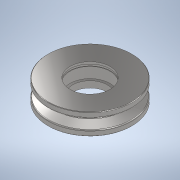
# Autodesk Inventor part: Pully
Saved by Autodesk Inventor 2021.1 (Build 251245010, 245A)
## iProperties
Created: 2025-09-16
Part Number: Pully
Material: Steel, Cast
Document SubType Name: Modeling
Designer: SD
Density: 7.85 g/cm^3
Appearance: Semi-Polished
Mass: 64.3377 g
Surface Area: 45.0663 cm^2
Volume: 8.19588 cm^3
Project: Automatic Tea Steeping mechanism
Length: 10.000 mm
BOM-Mass: 0.06434
BOM-Area: 0.005
Diameter: 40.000 mm
Author: SD
Title: Pully
Autodesk Inventor part; units mm, degrees
ref_plane "YZ Plane" through (0, 0, 0) normal (1, 0, 0) x (0, 1, 0)
ref_plane "XZ Plane" through (0, 0, 0) normal (0, 1, 0) x (-1, 0, 0)
ref_plane "XY Plane" through (0, 0, 0) normal (0, 0, 1) x (1, 0, 0)
sketch "Sketch1" plane through (0, 0, 0) normal (0, 0, 1) x (1, 0, 0)
  line L0 (0, 0) -> (0, -10) construction
  line L1 (8.25, -10) -> (20, -10)
  line L2 (20, -10) -> (20, -7.5)
  line L3 (20, -7.5) -> (15.3441, -5.75)
  line L4 (15.3441, -5.75) -> (15.3441, -4.25)
  line L5 (15.3441, -4.25) -> (20, -2.5)
  line L6 (20, -2.5) -> (20, 0)
  line L7 (20, 0) -> (9.5, 0)
  line L8 (9.5, 0) -> (9.5, -0.99)
  line L9 (9.5, -0.99) -> (9.8, -0.99)
  line L10 (9.8, -0.99) -> (9.8, -1.99)
  line L11 (9.8, -1.99) -> (9.5, -1.99)
  line L12 (9.5, -1.99) -> (9.5, -7)
  line L13 (9.5, -7) -> (8.25, -7)
  line L14 (8.25, -7) -> (8.25, -10)
  line L15 (15.3441, -5) -> (20.953, -5) construction
  dimension "d0" = 11.75
  dimension "d1" = 3
  dimension "Length" = 10
  dimension "d3" = 0.99
  dimension "d4" = 1
  dimension "d5" = 0.3
  dimension "d6" = 1.25
  dimension "d7" = 8.25
  dimension "d8" = 1.5
  dimension "d9" = 2.5
  dimension "d10" = 4.6559
  constraints: 32 end point, 8 perpendicular, 4 point on line, 2 equal length, 2 horizontal, 2 horizontal alignment, 1 midpoint, 1 parallel, 1 vertical
  measures "d0" distance of L1.start L1.end
  measures "d1" distance of L13.end L1.start
  measures "Length" distance between parallel lines of L7 L1
  measures "d3" distance of L7.end L8.end
  measures "d4" distance of L9.end L10.end
  measures "d5" distance of L8.end L9.end
  measures "d6" distance of L12.end L13.end
  measures "d7" distance between parallel lines of L14 L0
  measures "d8" distance of L3.end L4.end
  measures "d9" distance from line of L5.end L15
  measures "d10" distance between parallel lines of L6 L4
revolve "Revolution1" add sketch "Sketch1" angle 360 about axis through (0, 0, 0) along (0, -1, 0)
fillet "Fillet1" radius 0.5 4 edges at (-15.3441, -5.75, 0) (-15.3441, -4.25, 0) (-20, -7.5, 0) (-20, -2.5, 0)
chamfer "Chamfer1" distance 0.2 angle 45 2 edges at (-20, 0, 0) (-20, -10, 0)
equation "\"Diameter\" = 40"
body "Solid1"
